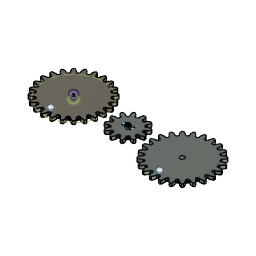
gearshuman (Autodesk Fusion 360 design; units mm, degrees)
description: Spur Gear; Module: 2.5; Num Teeth: 24; Pressure Angle: 20.0; Backlash: 0.00 mm
part number: 2026-02-21-14-46-09-125
Autodesk Fusion 360 part; units mm, degrees
(part 1 of 5)
sketch "Sketch1" plane through (0, 0, 0) normal (0, 0, 1) x (1, 0, 0)
sketch "Base Circle" plane through (0, 0, 0) normal (0, 0, 1) x (1, 0, 0)
  circle A0 centre (0, 0) radius 54.215
  circle A1 centre (0, 0) radius 2.6
sketch "Gear Tooth" plane through (0, 0, 0) normal (0, 0, 1) x (1, 0, 0)
  spline S0 degree 5 poles (56.1996, -4.5256) (56.225, -4.5277) (56.2758, -4.5311) (56.3519, -4.5344) (56.4536, -4.535) (56.5807, -4.5308) (56.708, -4.5231) (56.8353, -4.5131) (56.9627, -4.502) (57.0901, -4.49) (57.2175, -4.4772) (57.3449, -4.4633) (57.4722, -4.4478) (57.5996, -4.4307) (57.7269, -4.4118) (57.8543, -4.3913) (57.9815, -4.3694) (58.1088, -4.3463) (58.236, -4.3223) (58.3632, -4.2974) (58.4903, -4.2715) (58.6173, -4.2446) (58.7443, -4.2166) (58.8713, -4.1876) (58.9982, -4.1575) (59.125, -4.1264) (59.2517, -4.0943) (59.3784, -4.0613) (59.505, -4.0274) (59.6316, -3.9927) (59.758, -3.9571) (59.8844, -3.9206) (60.0107, -3.8833) (60.1369, -3.8452) (60.2631, -3.8061) (60.3891, -3.7663) (60.5151, -3.7256) (60.6409, -3.6842) (60.7667, -3.642) (60.8924, -3.599) (61.018, -3.5552) (61.1434, -3.5107) (61.2688, -3.4654) (61.3941, -3.4193) (61.5193, -3.3726) (61.6443, -3.3251) (61.7693, -3.2769) (61.8942, -3.2279) (62.0189, -3.1783) (62.1435, -3.1279) (62.268, -3.0769) (62.3924, -3.0252) (62.5167, -2.9728) (62.6409, -2.9197) (62.7649, -2.8659) (62.8888, -2.8115) (63.0126, -2.7564) (63.1363, -2.7007) (63.2598, -2.6443) (63.3833, -2.5872) (63.5065, -2.5295) (63.6297, -2.4712) (63.7527, -2.4122) (63.8756, -2.3527) (63.9984, -2.2925) (64.121, -2.2316) (64.2435, -2.1702) (64.3658, -2.1081) (64.488, -2.0455) (64.6101, -1.9822) (64.732, -1.9183) (64.8294, -1.8668) (64.9024, -1.8278) (64.9511, -1.8017) (64.9754, -1.7887) knots 0 0 0 0 0 0 0.01428571 0.02857143 0.04285714 0.05714286 0.07142857 0.08571429 0.1 0.11428571 0.12857143 0.14285714 0.15714286 0.17142857 0.18571429 0.2 0.21428571 0.22857143 0.24285714 0.25714286 0.27142857 0.28571429 0.3 0.31428571 0.32857143 0.34285714 0.35714286 0.37142857 0.38571429 0.4 0.41428571 0.42857143 0.44285714 0.45714286 0.47142857 0.48571429 0.5 0.51428571 0.52857143 0.54285714 0.55714286 0.57142857 0.58571429 0.6 0.61428571 0.62857143 0.64285714 0.65714286 0.67142857 0.68571429 0.7 0.71428571 0.72857143 0.74285714 0.75714286 0.77142857 0.78571429 0.8 0.81428571 0.82857143 0.84285714 0.85714286 0.87142857 0.88571429 0.9 0.91428571 0.92857143 0.94285714 0.95714286 0.97142857 0.98571429 1 1 1 1 1 1
  spline S1 degree 5 poles (56.1996, 4.5256) (56.225, 4.5277) (56.2758, 4.5311) (56.3519, 4.5344) (56.4536, 4.535) (56.5807, 4.5308) (56.708, 4.5231) (56.8353, 4.5131) (56.9627, 4.502) (57.0901, 4.49) (57.2175, 4.4772) (57.3449, 4.4633) (57.4722, 4.4478) (57.5996, 4.4307) (57.7269, 4.4118) (57.8543, 4.3913) (57.9815, 4.3694) (58.1088, 4.3463) (58.236, 4.3223) (58.3632, 4.2974) (58.4903, 4.2715) (58.6173, 4.2446) (58.7443, 4.2166) (58.8713, 4.1876) (58.9982, 4.1575) (59.125, 4.1264) (59.2517, 4.0943) (59.3784, 4.0613) (59.505, 4.0274) (59.6316, 3.9927) (59.758, 3.9571) (59.8844, 3.9206) (60.0107, 3.8833) (60.1369, 3.8452) (60.2631, 3.8061) (60.3891, 3.7663) (60.5151, 3.7256) (60.6409, 3.6842) (60.7667, 3.642) (60.8924, 3.599) (61.018, 3.5552) (61.1434, 3.5107) (61.2688, 3.4654) (61.3941, 3.4193) (61.5193, 3.3726) (61.6443, 3.3251) (61.7693, 3.2769) (61.8942, 3.2279) (62.0189, 3.1783) (62.1435, 3.1279) (62.268, 3.0769) (62.3924, 3.0252) (62.5167, 2.9728) (62.6409, 2.9197) (62.7649, 2.8659) (62.8888, 2.8115) (63.0126, 2.7564) (63.1363, 2.7007) (63.2598, 2.6443) (63.3833, 2.5872) (63.5065, 2.5295) (63.6297, 2.4712) (63.7527, 2.4122) (63.8756, 2.3527) (63.9984, 2.2925) (64.121, 2.2316) (64.2435, 2.1702) (64.3658, 2.1081) (64.488, 2.0455) (64.6101, 1.9822) (64.732, 1.9183) (64.8294, 1.8668) (64.9024, 1.8278) (64.9511, 1.8017) (64.9754, 1.7887) knots 0 0 0 0 0 0 0.01428571 0.02857143 0.04285714 0.05714286 0.07142857 0.08571429 0.1 0.11428571 0.12857143 0.14285714 0.15714286 0.17142857 0.18571429 0.2 0.21428571 0.22857143 0.24285714 0.25714286 0.27142857 0.28571429 0.3 0.31428571 0.32857143 0.34285714 0.35714286 0.37142857 0.38571429 0.4 0.41428571 0.42857143 0.44285714 0.45714286 0.47142857 0.48571429 0.5 0.51428571 0.52857143 0.54285714 0.55714286 0.57142857 0.58571429 0.6 0.61428571 0.62857143 0.64285714 0.65714286 0.67142857 0.68571429 0.7 0.71428571 0.72857143 0.74285714 0.75714286 0.77142857 0.78571429 0.8 0.81428571 0.82857143 0.84285714 0.85714286 0.87142857 0.88571429 0.9 0.91428571 0.92857143 0.94285714 0.95714286 0.97142857 0.98571429 1 1 1 1 1 1
  arc A0 (64.9754, -1.7887) -> (64.9754, 1.7887) centre (0, 0) ccw
  line L0 (54.0301, -4.3509) -> (56.1996, -4.5256)
  line L1 (54.0301, 4.3509) -> (56.1996, 4.5256)
  line L2 (54.0301, -4.3509) -> (54.0301, 4.3509)
  point P0 (56.8181, -4.5142)
  point P1 (57.4405, -4.4514)
  point P2 (58.0653, -4.3541)
  point P3 (58.6919, -4.228)
  point P4 (59.3197, -4.0765)
  point P5 (59.9483, -3.9016)
  point P6 (60.5776, -3.7049)
  point P7 (61.2071, -3.4876)
  point P8 (61.8366, -3.2504)
  point P9 (62.4659, -2.9941)
  point P10 (63.0946, -2.7193)
  point P11 (63.7226, -2.4266)
  point P12 (64.3496, -2.1162)
  point P13 (56.8181, 4.5142)
  point P14 (57.4405, 4.4514)
  point P15 (58.0653, 4.3541)
  point P16 (58.6919, 4.228)
  point P17 (59.3197, 4.0765)
  point P18 (59.9483, 3.9016)
  point P19 (60.5776, 3.7049)
  point P20 (61.2071, 3.4876)
  point P21 (61.8366, 3.2504)
  point P22 (62.4659, 2.9941)
  point P23 (63.0946, 2.7193)
  point P24 (63.7226, 2.4266)
  point P25 (64.3496, 2.1162)
sketch "Diametrial Pitch Circle" plane through (0, 0, 0) normal (0, 0, 1) x (1, 0, 0)
sketch "Base Circle (1)" plane through (0, 0, 0) normal (0, 0, 1) x (1, 0, 0)
  circle A0 centre (0, 0) radius 27.1075
  circle A1 centre (0, 0) radius 2.6
sketch "Gear Tooth (1)" plane through (0, 0, 0) normal (0, 0, 1) x (1, 0, 0)
  spline S0 degree 5 poles (28.0998, -2.2628) (28.1124, -2.2638) (28.1377, -2.2655) (28.1756, -2.2672) (28.2262, -2.2675) (28.2895, -2.2655) (28.3528, -2.2616) (28.4162, -2.2567) (28.4797, -2.2511) (28.5431, -2.2452) (28.6066, -2.2388) (28.67, -2.2319) (28.7335, -2.2242) (28.797, -2.2157) (28.8605, -2.2063) (28.9239, -2.1962) (28.9874, -2.1853) (29.0508, -2.1738) (29.1143, -2.1619) (29.1777, -2.1495) (29.2411, -2.1366) (29.3045, -2.1232) (29.3679, -2.1093) (29.4312, -2.0948) (29.4946, -2.0798) (29.5579, -2.0643) (29.6212, -2.0484) (29.6844, -2.0319) (29.7477, -2.015) (29.8109, -1.9977) (29.8741, -1.98) (29.9372, -1.9618) (30.0003, -1.9432) (30.0634, -1.9241) (30.1264, -1.9047) (30.1895, -1.8848) (30.2524, -1.8645) (30.3154, -1.8438) (30.3783, -1.8227) (30.4411, -1.8012) (30.504, -1.7794) (30.5667, -1.7571) (30.6295, -1.7345) (30.6922, -1.7115) (30.7548, -1.6881) (30.8174, -1.6644) (30.88, -1.6402) (30.9425, -1.6158) (31.005, -1.5909) (31.0674, -1.5658) (31.1297, -1.5402) (31.1921, -1.5143) (31.2543, -1.4881) (31.3165, -1.4615) (31.3787, -1.4346) (31.4408, -1.4073) (31.5029, -1.3797) (31.5649, -1.3518) (31.6268, -1.3236) (31.6887, -1.295) (31.7505, -1.2661) (31.8123, -1.2368) (31.874, -1.2073) (31.9356, -1.1774) (31.9972, -1.1472) (32.0588, -1.1167) (32.1202, -1.0858) (32.1816, -1.0547) (32.243, -1.0233) (32.3043, -0.9915) (32.3655, -0.9594) (32.4144, -0.9336) (32.4511, -0.914) (32.4755, -0.9009) (32.4877, -0.8943) knots 0 0 0 0 0 0 0.01428571 0.02857143 0.04285714 0.05714286 0.07142857 0.08571429 0.1 0.11428571 0.12857143 0.14285714 0.15714286 0.17142857 0.18571429 0.2 0.21428571 0.22857143 0.24285714 0.25714286 0.27142857 0.28571429 0.3 0.31428571 0.32857143 0.34285714 0.35714286 0.37142857 0.38571429 0.4 0.41428571 0.42857143 0.44285714 0.45714286 0.47142857 0.48571429 0.5 0.51428571 0.52857143 0.54285714 0.55714286 0.57142857 0.58571429 0.6 0.61428571 0.62857143 0.64285714 0.65714286 0.67142857 0.68571429 0.7 0.71428571 0.72857143 0.74285714 0.75714286 0.77142857 0.78571429 0.8 0.81428571 0.82857143 0.84285714 0.85714286 0.87142857 0.88571429 0.9 0.91428571 0.92857143 0.94285714 0.95714286 0.97142857 0.98571429 1 1 1 1 1 1
  spline S1 degree 5 poles (28.0998, 2.2628) (28.1124, 2.2638) (28.1377, 2.2655) (28.1756, 2.2672) (28.2262, 2.2675) (28.2895, 2.2655) (28.3528, 2.2616) (28.4162, 2.2567) (28.4797, 2.2511) (28.5431, 2.2452) (28.6066, 2.2388) (28.67, 2.2319) (28.7335, 2.2242) (28.797, 2.2157) (28.8605, 2.2063) (28.9239, 2.1962) (28.9874, 2.1853) (29.0508, 2.1738) (29.1143, 2.1619) (29.1777, 2.1495) (29.2411, 2.1366) (29.3045, 2.1232) (29.3679, 2.1093) (29.4312, 2.0948) (29.4946, 2.0798) (29.5579, 2.0643) (29.6212, 2.0484) (29.6844, 2.0319) (29.7477, 2.015) (29.8109, 1.9977) (29.8741, 1.98) (29.9372, 1.9618) (30.0003, 1.9432) (30.0634, 1.9241) (30.1264, 1.9047) (30.1895, 1.8848) (30.2524, 1.8645) (30.3154, 1.8438) (30.3783, 1.8227) (30.4411, 1.8012) (30.504, 1.7794) (30.5667, 1.7571) (30.6295, 1.7345) (30.6922, 1.7115) (30.7548, 1.6881) (30.8174, 1.6644) (30.88, 1.6402) (30.9425, 1.6158) (31.005, 1.5909) (31.0674, 1.5658) (31.1297, 1.5402) (31.1921, 1.5143) (31.2543, 1.4881) (31.3165, 1.4615) (31.3787, 1.4346) (31.4408, 1.4073) (31.5029, 1.3797) (31.5649, 1.3518) (31.6268, 1.3236) (31.6887, 1.295) (31.7505, 1.2661) (31.8123, 1.2368) (31.874, 1.2073) (31.9356, 1.1774) (31.9972, 1.1472) (32.0588, 1.1167) (32.1202, 1.0858) (32.1816, 1.0547) (32.243, 1.0233) (32.3043, 0.9915) (32.3655, 0.9594) (32.4144, 0.9336) (32.4511, 0.914) (32.4755, 0.9009) (32.4877, 0.8943) knots 0 0 0 0 0 0 0.01428571 0.02857143 0.04285714 0.05714286 0.07142857 0.08571429 0.1 0.11428571 0.12857143 0.14285714 0.15714286 0.17142857 0.18571429 0.2 0.21428571 0.22857143 0.24285714 0.25714286 0.27142857 0.28571429 0.3 0.31428571 0.32857143 0.34285714 0.35714286 0.37142857 0.38571429 0.4 0.41428571 0.42857143 0.44285714 0.45714286 0.47142857 0.48571429 0.5 0.51428571 0.52857143 0.54285714 0.55714286 0.57142857 0.58571429 0.6 0.61428571 0.62857143 0.64285714 0.65714286 0.67142857 0.68571429 0.7 0.71428571 0.72857143 0.74285714 0.75714286 0.77142857 0.78571429 0.8 0.81428571 0.82857143 0.84285714 0.85714286 0.87142857 0.88571429 0.9 0.91428571 0.92857143 0.94285714 0.95714286 0.97142857 0.98571429 1 1 1 1 1 1
  arc A0 (32.4877, -0.8943) -> (32.4877, 0.8943) centre (0, 0) ccw
  line L0 (27.0101, -2.1751) -> (28.0998, -2.2628)
  line L1 (27.0101, 2.1751) -> (28.0998, 2.2628)
  line L2 (27.0101, -2.1751) -> (27.0101, 2.1751)
  point P0 (28.4091, -2.2571)
  point P1 (28.7203, -2.2257)
  point P2 (29.0327, -2.177)
  point P3 (29.3459, -2.114)
  point P4 (29.6598, -2.0382)
  point P5 (29.9742, -1.9508)
  point P6 (30.2888, -1.8525)
  point P7 (30.6036, -1.7438)
  point P8 (30.9183, -1.6252)
  point P9 (31.2329, -1.4971)
  point P10 (31.5473, -1.3597)
  point P11 (31.8613, -1.2133)
  point P12 (32.1748, -1.0581)
  point P13 (28.4091, 2.2571)
  point P14 (28.7203, 2.2257)
  point P15 (29.0327, 2.177)
  point P16 (29.3459, 2.114)
  point P17 (29.6598, 2.0382)
  point P18 (29.9742, 1.9508)
  point P19 (30.2888, 1.8525)
  point P20 (30.6036, 1.7438)
  point P21 (30.9183, 1.6252)
  point P22 (31.2329, 1.4971)
  point P23 (31.5473, 1.3597)
  point P24 (31.8613, 1.2133)
  point P25 (32.1748, 1.0581)
sketch "Diametrial Pitch Circle (1)" plane through (0, 0, 0) normal (0, 0, 1) x (1, 0, 0)
sketch "Base Circle (2)" plane through (0, 0, 0) normal (0, 0, 1) x (1, 0, 0)
  circle A0 centre (0, 0) radius 27.1075
  circle A1 centre (0, 0) radius 2.6
sketch "Gear Tooth (2)" plane through (0, 0, 0) normal (0, 0, 1) x (1, 0, 0)
  spline S0 degree 5 poles (28.0998, -2.2628) (28.1124, -2.2638) (28.1377, -2.2655) (28.1756, -2.2672) (28.2262, -2.2675) (28.2895, -2.2655) (28.3528, -2.2616) (28.4162, -2.2567) (28.4797, -2.2511) (28.5431, -2.2452) (28.6066, -2.2388) (28.67, -2.2319) (28.7335, -2.2242) (28.797, -2.2157) (28.8605, -2.2063) (28.9239, -2.1962) (28.9874, -2.1853) (29.0508, -2.1738) (29.1143, -2.1619) (29.1777, -2.1495) (29.2411, -2.1366) (29.3045, -2.1232) (29.3679, -2.1093) (29.4312, -2.0948) (29.4946, -2.0798) (29.5579, -2.0643) (29.6212, -2.0484) (29.6844, -2.0319) (29.7477, -2.015) (29.8109, -1.9977) (29.8741, -1.98) (29.9372, -1.9618) (30.0003, -1.9432) (30.0634, -1.9241) (30.1264, -1.9047) (30.1895, -1.8848) (30.2524, -1.8645) (30.3154, -1.8438) (30.3783, -1.8227) (30.4411, -1.8012) (30.504, -1.7794) (30.5667, -1.7571) (30.6295, -1.7345) (30.6922, -1.7115) (30.7548, -1.6881) (30.8174, -1.6644) (30.88, -1.6402) (30.9425, -1.6158) (31.005, -1.5909) (31.0674, -1.5658) (31.1297, -1.5402) (31.1921, -1.5143) (31.2543, -1.4881) (31.3165, -1.4615) (31.3787, -1.4346) (31.4408, -1.4073) (31.5029, -1.3797) (31.5649, -1.3518) (31.6268, -1.3236) (31.6887, -1.295) (31.7505, -1.2661) (31.8123, -1.2368) (31.874, -1.2073) (31.9356, -1.1774) (31.9972, -1.1472) (32.0588, -1.1167) (32.1202, -1.0858) (32.1816, -1.0547) (32.243, -1.0233) (32.3043, -0.9915) (32.3655, -0.9594) (32.4144, -0.9336) (32.4511, -0.914) (32.4755, -0.9009) (32.4877, -0.8943) knots 0 0 0 0 0 0 0.01428571 0.02857143 0.04285714 0.05714286 0.07142857 0.08571429 0.1 0.11428571 0.12857143 0.14285714 0.15714286 0.17142857 0.18571429 0.2 0.21428571 0.22857143 0.24285714 0.25714286 0.27142857 0.28571429 0.3 0.31428571 0.32857143 0.34285714 0.35714286 0.37142857 0.38571429 0.4 0.41428571 0.42857143 0.44285714 0.45714286 0.47142857 0.48571429 0.5 0.51428571 0.52857143 0.54285714 0.55714286 0.57142857 0.58571429 0.6 0.61428571 0.62857143 0.64285714 0.65714286 0.67142857 0.68571429 0.7 0.71428571 0.72857143 0.74285714 0.75714286 0.77142857 0.78571429 0.8 0.81428571 0.82857143 0.84285714 0.85714286 0.87142857 0.88571429 0.9 0.91428571 0.92857143 0.94285714 0.95714286 0.97142857 0.98571429 1 1 1 1 1 1
  spline S1 degree 5 poles (28.0998, 2.2628) (28.1124, 2.2638) (28.1377, 2.2655) (28.1756, 2.2672) (28.2262, 2.2675) (28.2895, 2.2655) (28.3528, 2.2616) (28.4162, 2.2567) (28.4797, 2.2511) (28.5431, 2.2452) (28.6066, 2.2388) (28.67, 2.2319) (28.7335, 2.2242) (28.797, 2.2157) (28.8605, 2.2063) (28.9239, 2.1962) (28.9874, 2.1853) (29.0508, 2.1738) (29.1143, 2.1619) (29.1777, 2.1495) (29.2411, 2.1366) (29.3045, 2.1232) (29.3679, 2.1093) (29.4312, 2.0948) (29.4946, 2.0798) (29.5579, 2.0643) (29.6212, 2.0484) (29.6844, 2.0319) (29.7477, 2.015) (29.8109, 1.9977) (29.8741, 1.98) (29.9372, 1.9618) (30.0003, 1.9432) (30.0634, 1.9241) (30.1264, 1.9047) (30.1895, 1.8848) (30.2524, 1.8645) (30.3154, 1.8438) (30.3783, 1.8227) (30.4411, 1.8012) (30.504, 1.7794) (30.5667, 1.7571) (30.6295, 1.7345) (30.6922, 1.7115) (30.7548, 1.6881) (30.8174, 1.6644) (30.88, 1.6402) (30.9425, 1.6158) (31.005, 1.5909) (31.0674, 1.5658) (31.1297, 1.5402) (31.1921, 1.5143) (31.2543, 1.4881) (31.3165, 1.4615) (31.3787, 1.4346) (31.4408, 1.4073) (31.5029, 1.3797) (31.5649, 1.3518) (31.6268, 1.3236) (31.6887, 1.295) (31.7505, 1.2661) (31.8123, 1.2368) (31.874, 1.2073) (31.9356, 1.1774) (31.9972, 1.1472) (32.0588, 1.1167) (32.1202, 1.0858) (32.1816, 1.0547) (32.243, 1.0233) (32.3043, 0.9915) (32.3655, 0.9594) (32.4144, 0.9336) (32.4511, 0.914) (32.4755, 0.9009) (32.4877, 0.8943) knots 0 0 0 0 0 0 0.01428571 0.02857143 0.04285714 0.05714286 0.07142857 0.08571429 0.1 0.11428571 0.12857143 0.14285714 0.15714286 0.17142857 0.18571429 0.2 0.21428571 0.22857143 0.24285714 0.25714286 0.27142857 0.28571429 0.3 0.31428571 0.32857143 0.34285714 0.35714286 0.37142857 0.38571429 0.4 0.41428571 0.42857143 0.44285714 0.45714286 0.47142857 0.48571429 0.5 0.51428571 0.52857143 0.54285714 0.55714286 0.57142857 0.58571429 0.6 0.61428571 0.62857143 0.64285714 0.65714286 0.67142857 0.68571429 0.7 0.71428571 0.72857143 0.74285714 0.75714286 0.77142857 0.78571429 0.8 0.81428571 0.82857143 0.84285714 0.85714286 0.87142857 0.88571429 0.9 0.91428571 0.92857143 0.94285714 0.95714286 0.97142857 0.98571429 1 1 1 1 1 1
  arc A0 (32.4877, -0.8943) -> (32.4877, 0.8943) centre (0, 0) ccw
  line L0 (27.0101, -2.1751) -> (28.0998, -2.2628)
  line L1 (27.0101, 2.1751) -> (28.0998, 2.2628)
  line L2 (27.0101, -2.1751) -> (27.0101, 2.1751)
  point P0 (28.4091, -2.2571)
  point P1 (28.7203, -2.2257)
  point P2 (29.0327, -2.177)
  point P3 (29.3459, -2.114)
  point P4 (29.6598, -2.0382)
  point P5 (29.9742, -1.9508)
  point P6 (30.2888, -1.8525)
  point P7 (30.6036, -1.7438)
  point P8 (30.9183, -1.6252)
  point P9 (31.2329, -1.4971)
  point P10 (31.5473, -1.3597)
  point P11 (31.8613, -1.2133)
  point P12 (32.1748, -1.0581)
  point P13 (28.4091, 2.2571)
  point P14 (28.7203, 2.2257)
  point P15 (29.0327, 2.177)
  point P16 (29.3459, 2.114)
  point P17 (29.6598, 2.0382)
  point P18 (29.9742, 1.9508)
  point P19 (30.2888, 1.8525)
  point P20 (30.6036, 1.7438)
  point P21 (30.9183, 1.6252)
  point P22 (31.2329, 1.4971)
  point P23 (31.5473, 1.3597)
  point P24 (31.8613, 1.2133)
  point P25 (32.1748, 1.0581)
sketch "Diametrial Pitch Circle (2)" plane through (0, 0, 0) normal (0, 0, 1) x (1, 0, 0)
sketch "Base Circle (3)" plane through (0, 0, 0) normal (0, 0, 1) x (1, 0, 0)
  circle A0 centre (0, 0) radius 12.1075
  circle A1 centre (0, 0) radius 2.6
extrude "Extrude7" add sketch "Base Circle (3)" along normal blind 3.3 makes body 1
sketch "Gear Tooth (3)" plane through (0, 0, 0) normal (0, 0, 1) x (1, 0, 0)
  spline S0 degree 5 poles (13.9458, -2.0479) (13.9559, -2.0494) (13.9759, -2.052) (14.0061, -2.055) (14.0465, -2.0571) (14.0972, -2.0572) (14.1481, -2.0556) (14.199, -2.0528) (14.2501, -2.0495) (14.3011, -2.0457) (14.3522, -2.0415) (14.4034, -2.0367) (14.4546, -2.0311) (14.5058, -2.0247) (14.5571, -2.0173) (14.6084, -2.0092) (14.6597, -2.0003) (14.7111, -1.9908) (14.7624, -1.9808) (14.8137, -1.9703) (14.8651, -1.9594) (14.9164, -1.9479) (14.9678, -1.9358) (15.0191, -1.9232) (15.0705, -1.91) (15.1218, -1.8963) (15.1731, -1.882) (15.2244, -1.8673) (15.2757, -1.8521) (15.3269, -1.8365) (15.3781, -1.8204) (15.4293, -1.8038) (15.4805, -1.7868) (15.5316, -1.7693) (15.5827, -1.7513) (15.6338, -1.7329) (15.6848, -1.7141) (15.7358, -1.6948) (15.7868, -1.6751) (15.8377, -1.655) (15.8886, -1.6345) (15.9394, -1.6136) (15.9902, -1.5922) (16.0409, -1.5705) (16.0916, -1.5483) (16.1422, -1.5258) (16.1928, -1.5028) (16.2433, -1.4794) (16.2937, -1.4557) (16.3441, -1.4316) (16.3944, -1.4071) (16.4447, -1.3822) (16.4949, -1.3569) (16.545, -1.3313) (16.5951, -1.3053) (16.6451, -1.2789) (16.695, -1.2521) (16.7448, -1.225) (16.7946, -1.1975) (16.8443, -1.1697) (16.8939, -1.1415) (16.9435, -1.1129) (16.9929, -1.084) (17.0423, -1.0548) (17.0916, -1.0251) (17.1408, -0.9952) (17.1899, -0.9649) (17.239, -0.9343) (17.2879, -0.9033) (17.3368, -0.8719) (17.3856, -0.8403) (17.4245, -0.8147) (17.4537, -0.7953) (17.4731, -0.7824) (17.4828, -0.7759) knots 0 0 0 0 0 0 0.01428571 0.02857143 0.04285714 0.05714286 0.07142857 0.08571429 0.1 0.11428571 0.12857143 0.14285714 0.15714286 0.17142857 0.18571429 0.2 0.21428571 0.22857143 0.24285714 0.25714286 0.27142857 0.28571429 0.3 0.31428571 0.32857143 0.34285714 0.35714286 0.37142857 0.38571429 0.4 0.41428571 0.42857143 0.44285714 0.45714286 0.47142857 0.48571429 0.5 0.51428571 0.52857143 0.54285714 0.55714286 0.57142857 0.58571429 0.6 0.61428571 0.62857143 0.64285714 0.65714286 0.67142857 0.68571429 0.7 0.71428571 0.72857143 0.74285714 0.75714286 0.77142857 0.78571429 0.8 0.81428571 0.82857143 0.84285714 0.85714286 0.87142857 0.88571429 0.9 0.91428571 0.92857143 0.94285714 0.95714286 0.97142857 0.98571429 1 1 1 1 1 1
  spline S1 degree 5 poles (13.9458, 2.0479) (13.9559, 2.0494) (13.9759, 2.052) (14.0061, 2.055) (14.0465, 2.0571) (14.0972, 2.0572) (14.1481, 2.0556) (14.199, 2.0528) (14.2501, 2.0495) (14.3011, 2.0457) (14.3522, 2.0415) (14.4034, 2.0367) (14.4546, 2.0311) (14.5058, 2.0247) (14.5571, 2.0173) (14.6084, 2.0092) (14.6597, 2.0003) (14.7111, 1.9908) (14.7624, 1.9808) (14.8137, 1.9703) (14.8651, 1.9594) (14.9164, 1.9479) (14.9678, 1.9358) (15.0191, 1.9232) (15.0705, 1.91) (15.1218, 1.8963) (15.1731, 1.882) (15.2244, 1.8673) (15.2757, 1.8521) (15.3269, 1.8365) (15.3781, 1.8204) (15.4293, 1.8038) (15.4805, 1.7868) (15.5316, 1.7693) (15.5827, 1.7513) (15.6338, 1.7329) (15.6848, 1.7141) (15.7358, 1.6948) (15.7868, 1.6751) (15.8377, 1.655) (15.8886, 1.6345) (15.9394, 1.6136) (15.9902, 1.5922) (16.0409, 1.5705) (16.0916, 1.5483) (16.1422, 1.5258) (16.1928, 1.5028) (16.2433, 1.4794) (16.2937, 1.4557) (16.3441, 1.4316) (16.3944, 1.4071) (16.4447, 1.3822) (16.4949, 1.3569) (16.545, 1.3313) (16.5951, 1.3053) (16.6451, 1.2789) (16.695, 1.2521) (16.7448, 1.225) (16.7946, 1.1975) (16.8443, 1.1697) (16.8939, 1.1415) (16.9435, 1.1129) (16.9929, 1.084) (17.0423, 1.0548) (17.0916, 1.0251) (17.1408, 0.9952) (17.1899, 0.9649) (17.239, 0.9343) (17.2879, 0.9033) (17.3368, 0.8719) (17.3856, 0.8403) (17.4245, 0.8147) (17.4537, 0.7953) (17.4731, 0.7824) (17.4828, 0.7759) knots 0 0 0 0 0 0 0.01428571 0.02857143 0.04285714 0.05714286 0.07142857 0.08571429 0.1 0.11428571 0.12857143 0.14285714 0.15714286 0.17142857 0.18571429 0.2 0.21428571 0.22857143 0.24285714 0.25714286 0.27142857 0.28571429 0.3 0.31428571 0.32857143 0.34285714 0.35714286 0.37142857 0.38571429 0.4 0.41428571 0.42857143 0.44285714 0.45714286 0.47142857 0.48571429 0.5 0.51428571 0.52857143 0.54285714 0.55714286 0.57142857 0.58571429 0.6 0.61428571 0.62857143 0.64285714 0.65714286 0.67142857 0.68571429 0.7 0.71428571 0.72857143 0.74285714 0.75714286 0.77142857 0.78571429 0.8 0.81428571 0.82857143 0.84285714 0.85714286 0.87142857 0.88571429 0.9 0.91428571 0.92857143 0.94285714 0.95714286 0.97142857 0.98571429 1 1 1 1 1 1
  arc A0 (17.4828, -0.7759) -> (17.4828, 0.7759) centre (0, 0) ccw
  line L0 (11.9691, -1.7576) -> (13.9458, -2.0479)
  line L1 (11.9691, 1.7576) -> (13.9458, 2.0479)
  line L2 (11.9691, -1.7576) -> (11.9691, 1.7576)
  point P0 (14.1908, -2.0531)
  point P1 (14.4394, -2.0327)
  point P2 (14.6902, -1.9946)
  point P3 (14.9425, -1.9417)
  point P4 (15.196, -1.8754)
  point P5 (15.4504, -1.7967)
  point P6 (15.7053, -1.7063)
  point P7 (15.9604, -1.6047)
  point P8 (16.2156, -1.4922)
  point P9 (16.4704, -1.3692)
  point P10 (16.7248, -1.2358)
  point P11 (16.9785, -1.0924)
  point P12 (17.2312, -0.939)
  point P13 (14.1908, 2.0531)
  point P14 (14.4394, 2.0327)
  point P15 (14.6902, 1.9946)
  point P16 (14.9425, 1.9417)
  point P17 (15.196, 1.8754)
  point P18 (15.4504, 1.7967)
  point P19 (15.7053, 1.7063)
  point P20 (15.9604, 1.6047)
  point P21 (16.2156, 1.4922)
  point P22 (16.4704, 1.3692)
  point P23 (16.7248, 1.2358)
  point P24 (16.9785, 1.0924)
  point P25 (17.2312, 0.939)
extrude "Extrude8" add sketch "Gear Tooth (3)" along normal blind 3.3 bodies 1
fillet "Fillet4" radius 1 2 edges at (11.979, -1.7591, 1.65) (11.979, 1.7591, 1.65) on bodies 1
pattern_circular "C-Pattern4" count 12 over 360 about axis through (0, 0, 0) along (0, 0, 1) of "Extrude8", "Fillet4"
sketch "Diametrial Pitch Circle (3)" plane through (0, 0, 0) normal (0, 0, 1) x (1, 0, 0)
move_body "Move2" bodies 1 to x (1, 0, 0) y (0, 1, 0) z (0, 0, 1) at (50, 0, 0)
move_body "Move4" bodies 1 to x (1, 0, 0) y (0, 1, 0) z (0, 0, 1) at (5, 0, 0)
sketch "Base Circle (4)" plane through (0, 0, 0) normal (0, 0, 1) x (1, 0, 0)
  circle A0 centre (0, 0) radius 27.1075
  circle A1 centre (0, 0) radius 2.25
extrude "Extrude9" add sketch "Base Circle (4)" along normal blind 3.3 separate body makes body 2
sketch "Gear Tooth (4)" plane through (0, 0, 0) normal (0, 0, 1) x (1, 0, 0)
  spline S0 degree 5 poles (28.0998, -2.2628) (28.1124, -2.2638) (28.1377, -2.2655) (28.1756, -2.2672) (28.2262, -2.2675) (28.2895, -2.2655) (28.3528, -2.2616) (28.4162, -2.2567) (28.4797, -2.2511) (28.5431, -2.2452) (28.6066, -2.2388) (28.67, -2.2319) (28.7335, -2.2242) (28.797, -2.2157) (28.8605, -2.2063) (28.9239, -2.1962) (28.9874, -2.1853) (29.0508, -2.1738) (29.1143, -2.1619) (29.1777, -2.1495) (29.2411, -2.1366) (29.3045, -2.1232) (29.3679, -2.1093) (29.4312, -2.0948) (29.4946, -2.0798) (29.5579, -2.0643) (29.6212, -2.0484) (29.6844, -2.0319) (29.7477, -2.015) (29.8109, -1.9977) (29.8741, -1.98) (29.9372, -1.9618) (30.0003, -1.9432) (30.0634, -1.9241) (30.1264, -1.9047) (30.1895, -1.8848) (30.2524, -1.8645) (30.3154, -1.8438) (30.3783, -1.8227) (30.4411, -1.8012) (30.504, -1.7794) (30.5667, -1.7571) (30.6295, -1.7345) (30.6922, -1.7115) (30.7548, -1.6881) (30.8174, -1.6644) (30.88, -1.6402) (30.9425, -1.6158) (31.005, -1.5909) (31.0674, -1.5658) (31.1297, -1.5402) (31.1921, -1.5143) (31.2543, -1.4881) (31.3165, -1.4615) (31.3787, -1.4346) (31.4408, -1.4073) (31.5029, -1.3797) (31.5649, -1.3518) (31.6268, -1.3236) (31.6887, -1.295) (31.7505, -1.2661) (31.8123, -1.2368) (31.874, -1.2073) (31.9356, -1.1774) (31.9972, -1.1472) (32.0588, -1.1167) (32.1202, -1.0858) (32.1816, -1.0547) (32.243, -1.0233) (32.3043, -0.9915) (32.3655, -0.9594) (32.4144, -0.9336) (32.4511, -0.914) (32.4755, -0.9009) (32.4877, -0.8943) knots 0 0 0 0 0 0 0.01428571 0.02857143 0.04285714 0.05714286 0.07142857 0.08571429 0.1 0.11428571 0.12857143 0.14285714 0.15714286 0.17142857 0.18571429 0.2 0.21428571 0.22857143 0.24285714 0.25714286 0.27142857 0.28571429 0.3 0.31428571 0.32857143 0.34285714 0.35714286 0.37142857 0.38571429 0.4 0.41428571 0.42857143 0.44285714 0.45714286 0.47142857 0.48571429 0.5 0.51428571 0.52857143 0.54285714 0.55714286 0.57142857 0.58571429 0.6 0.61428571 0.62857143 0.64285714 0.65714286 0.67142857 0.68571429 0.7 0.71428571 0.72857143 0.74285714 0.75714286 0.77142857 0.78571429 0.8 0.81428571 0.82857143 0.84285714 0.85714286 0.87142857 0.88571429 0.9 0.91428571 0.92857143 0.94285714 0.95714286 0.97142857 0.98571429 1 1 1 1 1 1
  spline S1 degree 5 poles (28.0998, 2.2628) (28.1124, 2.2638) (28.1377, 2.2655) (28.1756, 2.2672) (28.2262, 2.2675) (28.2895, 2.2655) (28.3528, 2.2616) (28.4162, 2.2567) (28.4797, 2.2511) (28.5431, 2.2452) (28.6066, 2.2388) (28.67, 2.2319) (28.7335, 2.2242) (28.797, 2.2157) (28.8605, 2.2063) (28.9239, 2.1962) (28.9874, 2.1853) (29.0508, 2.1738) (29.1143, 2.1619) (29.1777, 2.1495) (29.2411, 2.1366) (29.3045, 2.1232) (29.3679, 2.1093) (29.4312, 2.0948) (29.4946, 2.0798) (29.5579, 2.0643) (29.6212, 2.0484) (29.6844, 2.0319) (29.7477, 2.015) (29.8109, 1.9977) (29.8741, 1.98) (29.9372, 1.9618) (30.0003, 1.9432) (30.0634, 1.9241) (30.1264, 1.9047) (30.1895, 1.8848) (30.2524, 1.8645) (30.3154, 1.8438) (30.3783, 1.8227) (30.4411, 1.8012) (30.504, 1.7794) (30.5667, 1.7571) (30.6295, 1.7345) (30.6922, 1.7115) (30.7548, 1.6881) (30.8174, 1.6644) (30.88, 1.6402) (30.9425, 1.6158) (31.005, 1.5909) (31.0674, 1.5658) (31.1297, 1.5402) (31.1921, 1.5143) (31.2543, 1.4881) (31.3165, 1.4615) (31.3787, 1.4346) (31.4408, 1.4073) (31.5029, 1.3797) (31.5649, 1.3518) (31.6268, 1.3236) (31.6887, 1.295) (31.7505, 1.2661) (31.8123, 1.2368) (31.874, 1.2073) (31.9356, 1.1774) (31.9972, 1.1472) (32.0588, 1.1167) (32.1202, 1.0858) (32.1816, 1.0547) (32.243, 1.0233) (32.3043, 0.9915) (32.3655, 0.9594) (32.4144, 0.9336) (32.4511, 0.914) (32.4755, 0.9009) (32.4877, 0.8943) knots 0 0 0 0 0 0 0.01428571 0.02857143 0.04285714 0.05714286 0.07142857 0.08571429 0.1 0.11428571 0.12857143 0.14285714 0.15714286 0.17142857 0.18571429 0.2 0.21428571 0.22857143 0.24285714 0.25714286 0.27142857 0.28571429 0.3 0.31428571 0.32857143 0.34285714 0.35714286 0.37142857 0.38571429 0.4 0.41428571 0.42857143 0.44285714 0.45714286 0.47142857 0.48571429 0.5 0.51428571 0.52857143 0.54285714 0.55714286 0.57142857 0.58571429 0.6 0.61428571 0.62857143 0.64285714 0.65714286 0.67142857 0.68571429 0.7 0.71428571 0.72857143 0.74285714 0.75714286 0.77142857 0.78571429 0.8 0.81428571 0.82857143 0.84285714 0.85714286 0.87142857 0.88571429 0.9 0.91428571 0.92857143 0.94285714 0.95714286 0.97142857 0.98571429 1 1 1 1 1 1
  arc A0 (32.4877, -0.8943) -> (32.4877, 0.8943) centre (0, 0) ccw
  line L0 (27.0101, -2.1751) -> (28.0998, -2.2628)
  line L1 (27.0101, 2.1751) -> (28.0998, 2.2628)
  line L2 (27.0101, -2.1751) -> (27.0101, 2.1751)
  point P0 (28.4091, -2.2571)
  point P1 (28.7203, -2.2257)
  point P2 (29.0327, -2.177)
  point P3 (29.3459, -2.114)
  point P4 (29.6598, -2.0382)
  point P5 (29.9742, -1.9508)
  point P6 (30.2888, -1.8525)
  point P7 (30.6036, -1.7438)
  point P8 (30.9183, -1.6252)
  point P9 (31.2329, -1.4971)
  point P10 (31.5473, -1.3597)
  point P11 (31.8613, -1.2133)
  point P12 (32.1748, -1.0581)
  point P13 (28.4091, 2.2571)
  point P14 (28.7203, 2.2257)
  point P15 (29.0327, 2.177)
  point P16 (29.3459, 2.114)
  point P17 (29.6598, 2.0382)
  point P18 (29.9742, 1.9508)
  point P19 (30.2888, 1.8525)
  point P20 (30.6036, 1.7438)
  point P21 (30.9183, 1.6252)
  point P22 (31.2329, 1.4971)
  point P23 (31.5473, 1.3597)
  point P24 (31.8613, 1.2133)
  point P25 (32.1748, 1.0581)
extrude "Extrude10" add sketch "Gear Tooth (4)" along normal blind 3.3 bodies 2
fillet "Fillet5" radius 1 2 edges at (27.02, -2.1759, 1.65) (27.02, 2.1759, 1.65) on bodies 2
pattern_circular "C-Pattern5" count 24 over 360 about axis through (0, 0, 0) along (0, 0, 1) of "Extrude10", "Fillet5"
sketch "Diametrial Pitch Circle (4)" plane through (0, 0, 0) normal (0, 0, 1) x (1, 0, 0)
  circle A0 centre (0, 0) radius 30 construction
sketch "Base Circle (5)" plane through (0, 0, 0) normal (0, 0, 1) x (1, 0, 0)
  circle A0 centre (0, 0) radius 27.1075
  circle A1 centre (0, 0) radius 2.25
extrude "Extrude11" add sketch "Base Circle (5)" along normal blind 3.3 separate body makes body 3
sketch "Gear Tooth (5)" plane through (0, 0, 0) normal (0, 0, 1) x (1, 0, 0)
  spline S0 degree 5 poles (28.0998, -2.2628) (28.1124, -2.2638) (28.1377, -2.2655) (28.1756, -2.2672) (28.2262, -2.2675) (28.2895, -2.2655) (28.3528, -2.2616) (28.4162, -2.2567) (28.4797, -2.2511) (28.5431, -2.2452) (28.6066, -2.2388) (28.67, -2.2319) (28.7335, -2.2242) (28.797, -2.2157) (28.8605, -2.2063) (28.9239, -2.1962) (28.9874, -2.1853) (29.0508, -2.1738) (29.1143, -2.1619) (29.1777, -2.1495) (29.2411, -2.1366) (29.3045, -2.1232) (29.3679, -2.1093) (29.4312, -2.0948) (29.4946, -2.0798) (29.5579, -2.0643) (29.6212, -2.0484) (29.6844, -2.0319) (29.7477, -2.015) (29.8109, -1.9977) (29.8741, -1.98) (29.9372, -1.9618) (30.0003, -1.9432) (30.0634, -1.9241) (30.1264, -1.9047) (30.1895, -1.8848) (30.2524, -1.8645) (30.3154, -1.8438) (30.3783, -1.8227) (30.4411, -1.8012) (30.504, -1.7794) (30.5667, -1.7571) (30.6295, -1.7345) (30.6922, -1.7115) (30.7548, -1.6881) (30.8174, -1.6644) (30.88, -1.6402) (30.9425, -1.6158) (31.005, -1.5909) (31.0674, -1.5658) (31.1297, -1.5402) (31.1921, -1.5143) (31.2543, -1.4881) (31.3165, -1.4615) (31.3787, -1.4346) (31.4408, -1.4073) (31.5029, -1.3797) (31.5649, -1.3518) (31.6268, -1.3236) (31.6887, -1.295) (31.7505, -1.2661) (31.8123, -1.2368) (31.874, -1.2073) (31.9356, -1.1774) (31.9972, -1.1472) (32.0588, -1.1167) (32.1202, -1.0858) (32.1816, -1.0547) (32.243, -1.0233) (32.3043, -0.9915) (32.3655, -0.9594) (32.4144, -0.9336) (32.4511, -0.914) (32.4755, -0.9009) (32.4877, -0.8943) knots 0 0 0 0 0 0 0.01428571 0.02857143 0.04285714 0.05714286 0.07142857 0.08571429 0.1 0.11428571 0.12857143 0.14285714 0.15714286 0.17142857 0.18571429 0.2 0.21428571 0.22857143 0.24285714 0.25714286 0.27142857 0.28571429 0.3 0.31428571 0.32857143 0.34285714 0.35714286 0.37142857 0.38571429 0.4 0.41428571 0.42857143 0.44285714 0.45714286 0.47142857 0.48571429 0.5 0.51428571 0.52857143 0.54285714 0.55714286 0.57142857 0.58571429 0.6 0.61428571 0.62857143 0.64285714 0.65714286 0.67142857 0.68571429 0.7 0.71428571 0.72857143 0.74285714 0.75714286 0.77142857 0.78571429 0.8 0.81428571 0.82857143 0.84285714 0.85714286 0.87142857 0.88571429 0.9 0.91428571 0.92857143 0.94285714 0.95714286 0.97142857 0.98571429 1 1 1 1 1 1
  spline S1 degree 5 poles (28.0998, 2.2628) (28.1124, 2.2638) (28.1377, 2.2655) (28.1756, 2.2672) (28.2262, 2.2675) (28.2895, 2.2655) (28.3528, 2.2616) (28.4162, 2.2567) (28.4797, 2.2511) (28.5431, 2.2452) (28.6066, 2.2388) (28.67, 2.2319) (28.7335, 2.2242) (28.797, 2.2157) (28.8605, 2.2063) (28.9239, 2.1962) (28.9874, 2.1853) (29.0508, 2.1738) (29.1143, 2.1619) (29.1777, 2.1495) (29.2411, 2.1366) (29.3045, 2.1232) (29.3679, 2.1093) (29.4312, 2.0948) (29.4946, 2.0798) (29.5579, 2.0643) (29.6212, 2.0484) (29.6844, 2.0319) (29.7477, 2.015) (29.8109, 1.9977) (29.8741, 1.98) (29.9372, 1.9618) (30.0003, 1.9432) (30.0634, 1.9241) (30.1264, 1.9047) (30.1895, 1.8848) (30.2524, 1.8645) (30.3154, 1.8438) (30.3783, 1.8227) (30.4411, 1.8012) (30.504, 1.7794) (30.5667, 1.7571) (30.6295, 1.7345) (30.6922, 1.7115) (30.7548, 1.6881) (30.8174, 1.6644) (30.88, 1.6402) (30.9425, 1.6158) (31.005, 1.5909) (31.0674, 1.5658) (31.1297, 1.5402) (31.1921, 1.5143) (31.2543, 1.4881) (31.3165, 1.4615) (31.3787, 1.4346) (31.4408, 1.4073) (31.5029, 1.3797) (31.5649, 1.3518) (31.6268, 1.3236) (31.6887, 1.295) (31.7505, 1.2661) (31.8123, 1.2368) (31.874, 1.2073) (31.9356, 1.1774) (31.9972, 1.1472) (32.0588, 1.1167) (32.1202, 1.0858) (32.1816, 1.0547) (32.243, 1.0233) (32.3043, 0.9915) (32.3655, 0.9594) (32.4144, 0.9336) (32.4511, 0.914) (32.4755, 0.9009) (32.4877, 0.8943) knots 0 0 0 0 0 0 0.01428571 0.02857143 0.04285714 0.05714286 0.07142857 0.08571429 0.1 0.11428571 0.12857143 0.14285714 0.15714286 0.17142857 0.18571429 0.2 0.21428571 0.22857143 0.24285714 0.25714286 0.27142857 0.28571429 0.3 0.31428571 0.32857143 0.34285714 0.35714286 0.37142857 0.38571429 0.4 0.41428571 0.42857143 0.44285714 0.45714286 0.47142857 0.48571429 0.5 0.51428571 0.52857143 0.54285714 0.55714286 0.57142857 0.58571429 0.6 0.61428571 0.62857143 0.64285714 0.65714286 0.67142857 0.68571429 0.7 0.71428571 0.72857143 0.74285714 0.75714286 0.77142857 0.78571429 0.8 0.81428571 0.82857143 0.84285714 0.85714286 0.87142857 0.88571429 0.9 0.91428571 0.92857143 0.94285714 0.95714286 0.97142857 0.98571429 1 1 1 1 1 1
  arc A0 (32.4877, -0.8943) -> (32.4877, 0.8943) centre (0, 0) ccw
  line L0 (27.0101, -2.1751) -> (28.0998, -2.2628)
  line L1 (27.0101, 2.1751) -> (28.0998, 2.2628)
  line L2 (27.0101, -2.1751) -> (27.0101, 2.1751)
  point P0 (28.4091, -2.2571)
  point P1 (28.7203, -2.2257)
  point P2 (29.0327, -2.177)
  point P3 (29.3459, -2.114)
  point P4 (29.6598, -2.0382)
  point P5 (29.9742, -1.9508)
  point P6 (30.2888, -1.8525)
  point P7 (30.6036, -1.7438)
  point P8 (30.9183, -1.6252)
  point P9 (31.2329, -1.4971)
  point P10 (31.5473, -1.3597)
  point P11 (31.8613, -1.2133)
  point P12 (32.1748, -1.0581)
  point P13 (28.4091, 2.2571)
  point P14 (28.7203, 2.2257)
  point P15 (29.0327, 2.177)
  point P16 (29.3459, 2.114)
  point P17 (29.6598, 2.0382)
  point P18 (29.9742, 1.9508)
  point P19 (30.2888, 1.8525)
  point P20 (30.6036, 1.7438)
  point P21 (30.9183, 1.6252)
  point P22 (31.2329, 1.4971)
  point P23 (31.5473, 1.3597)
  point P24 (31.8613, 1.2133)
  point P25 (32.1748, 1.0581)
extrude "Extrude12" add sketch "Gear Tooth (5)" along normal blind 3.3 bodies 3
fillet "Fillet6" radius 1 2 edges at (27.02, -2.1759, 1.65) (27.02, 2.1759, 1.65) on bodies 3
pattern_circular "C-Pattern6" count 24 over 360 about axis through (0, 0, 0) along (0, 0, 1) of "Extrude12", "Fillet6"
sketch "Diametrial Pitch Circle (5)" plane through (0, 0, 0) normal (0, 0, 1) x (1, 0, 0)
  circle A0 centre (0, 0) radius 30 construction
move_body "Move5" bodies 3 to x (1, 0, 0) y (0, 1, 0) z (0, 0, 1) at (110, 0, 0)